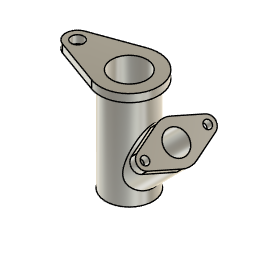
exercise08 (Autodesk Fusion 360 design; units mm, degrees)
Autodesk Fusion 360 part; units mm, degrees
note: some values were not read from the file. Chosen so that the rebuilt part matches the saved one: where a step ends.
sketch "草图1" plane through (0, 0, 0) normal (0, 1, 0) x (1, 0, 0)
  line L0 (60, 0) -> (60, -241)
  line L1 (60, -241) -> (75, -241)
  line L2 (75, -241) -> (75, -261)
  line L3 (75, -261) -> (45, -261)
  line L4 (45, -261) -> (45, 0)
  line L5 (45, 0) -> (60, 0)
  line L6 (0, -85) -> (0, 25) construction
  dimension "d1" = 75
  dimension "d2" = 261
  dimension "d3" = 20
  dimension "d4" = 45
  dimension "d5" = 60
  constraint vertical L0
  constraint perpendicular L0 L1
  constraint perpendicular L1 L2
  constraint perpendicular L2 L3
  constraint perpendicular L3 L4
  constraint perpendicular L0 L5
  constraint vertical L6
  constraint collinear origin L0.start L4.end
  measures "d1" distance of L2.end L6
  measures "d2" distance of L3 L5
  measures "d3" distance of L1.end L2.end
  measures "d4" distance of origin L4.end
  measures "d5" distance of origin L0.start
revolve "旋转1" add sketch "草图1" angle 360 about axis through (0, 0, 85) along (0, 0, -1) makes body 1
sketch "草图2" plane through (0, 0, 261) normal (0, 0, 1) x (-1, 0, 0)
  circle A0 centre (0, 0) radius 75
  circle A1 centre (0, 0) radius 45
  circle A2 centre (0, 0) radius 75
  circle A3 centre (132, 0) radius 16
  line L0 (142.2273, -28.2029) -> (25.5682, -70.5072)
  line L1 (25.5682, 70.5072) -> (142.2273, 28.2029)
  arc A4 (142.2273, -28.2029) -> (142.2273, 28.2029) centre (132, 0) ccw
  point P0 (-75, 0)
  dimension "d7" = 150
  dimension "d8" = 32
  dimension "d9" = 60
  dimension "d10" = 132
  constraint coincident A0.centre A1.centre
  constraint concentric A3 A4
  constraint coincident A2 L0.end
  constraint coincident A2 L1.start
  constraint collinear A0.centre A3.centre P0
  constraint tangent L0 A4
  constraint tangent A2 L0
  constraint tangent A2 L1
  constraint tangent L1 A4
  measures "d7" diameter of A2
  measures "d8" diameter of A3
  measures "d9" diameter of A4
  measures "d10" distance of A0.centre A3.centre
extrude "拉伸1" add sketch "草图2" against normal blind 20 contours A0 A2 L0 L1 A4 bodies 1
ref_plane "工作平面2" through (0, 12.125, 0) normal (0.707107, 0, 0.707107) x (0, 1, 0)
ref_plane "工作平面3" through (148.4924, 12.125, 148.4924) normal (0.707107, 0, 0.707107) x (0, 1, 0)
sketch "草图3" plane through (148.4924, 0, 148.4924) normal (0.707107, 0, 0.707107) x (0, 1, 0)
  circle A0 centre (-80, 0) radius 10
  circle A1 centre (80, 0) radius 10
  line L0 (-87.5, 18.5405) -> (-18.75, 46.3512)
  line L1 (18.75, 46.3512) -> (87.5, 18.5405)
  line L2 (87.5, -18.5405) -> (18.75, -46.3512)
  line L3 (-18.75, -46.3512) -> (-87.5, -18.5405)
  line L4 (0, 125.2902) -> (0, -120) construction
  circle A2 centre (0, 0) radius 30
  arc A3 (-87.5, 18.5405) -> (-87.5, -18.5405) centre (-80, 0) ccw
  arc A4 (-18.75, -46.3512) -> (18.75, -46.3512) centre (0, 0) ccw
  arc A5 (18.75, 46.3512) -> (-18.75, 46.3512) centre (0, 0) ccw
  arc A6 (87.5, -18.5405) -> (87.5, 18.5405) centre (80, 0) ccw
  dimension "d16" = 160
  dimension "d17" = 40
  dimension "d18" = 20
  dimension "d19" = 100
  dimension "d20" = 60
  constraint coincident A2.centre A4.centre
  constraint concentric A0 A3
  constraint concentric A1 A6
  constraint coincident L0.start A3
  constraint tangent L0 A4
  constraint coincident L1.start A4
  constraint tangent L2 A6
  constraint equal A3 A6
  constraint equal A0 A1
  constraint vertical L4
  constraint collinear A2.centre A1.centre A0.centre
  constraint symmetric L4 A3 A6
  constraint tangent L3 A4
  constraint tangent L1 A4
  constraint tangent L1 A6
  constraint tangent L2 A4
  constraint tangent L3 A3
  constraint coincident L0 A3.start
  constraint concentric A4 A5
  constraint equal L0 L1
  measures "d16" distance of A1.centre A0.centre
  measures "d17" diameter of A6
  measures "d18" diameter of A1
  measures "d19" diameter of A4
  measures "d20" diameter of A2
extrude "拉伸2" add sketch "草图3" against normal blind 20 separate body makes body 2
move_body "移动1" bodies 2 to x (1, 0, 0) y (0, 1, 0) z (0, 0, 1) at (-14.1421, 0, -14.1421)
move_body "移动2" bodies 2 to x (1, 0, 0) y (0, 1, 0) z (0, 0, 1) at (-134.3503, 0, -134.3503)
move_body "移动3" bodies 2 to x (1, 0, 0) y (0, 1, 0) z (0, 0, 1) at (120, 0, 160)
sketch "草图4" plane through (140, 0, 140) normal (0.707107, 0, 0.707107) x (0, 1, 0)
  circle A0 centre (-80, 28.2843) radius 10
  circle A1 centre (80, 28.2843) radius 10
  circle A2 centre (0, 28.2843) radius 30
  arc A3 (-18.75, -18.067) -> (18.75, -18.067) centre (0, 28.2843) ccw
  line L0 (18.75, -18.067) -> (87.5, 9.7438)
  arc A4 (87.5, 9.7438) -> (87.5, 46.8248) centre (80, 28.2843) ccw
  line L1 (87.5, 46.8248) -> (18.75, 74.6355)
  arc A5 (18.75, 74.6355) -> (-18.75, 74.6355) centre (0, 28.2843) ccw
  line L2 (-18.75, 74.6355) -> (-87.5, 46.8248)
  arc A6 (-87.5, 46.8248) -> (-87.5, 9.7438) centre (-80, 28.2843) ccw
  line L3 (-87.5, 9.7438) -> (-18.75, -18.067)
  line L4 (-80, 28.2843) -> (80, 28.2843)
  circle A7 centre (0, 28.2843) radius 30
  circle A8 centre (0, 28.2843) radius 50
  constraint coincident A0.centre A6.centre
  constraint coincident A1.centre A4.centre
  constraint concentric A2 A7
  constraint concentric A7 A8
extrude "拉伸3" add sketch "草图4" along normal up to near side of body 1 contours A2 A3 L4 A7 A8 | A2 A5 L4 A7 A8 bodies 1 2
extrude "拉伸4" cut sketch "草图4" along normal up to surface contours A2 L4 A7 | A2 L4 A7 end surface at (44.9441, 2.2431, 174) on bodies 1 bodies 1
equation "d1 = ( 150 / 2 ) * 1 mm"
